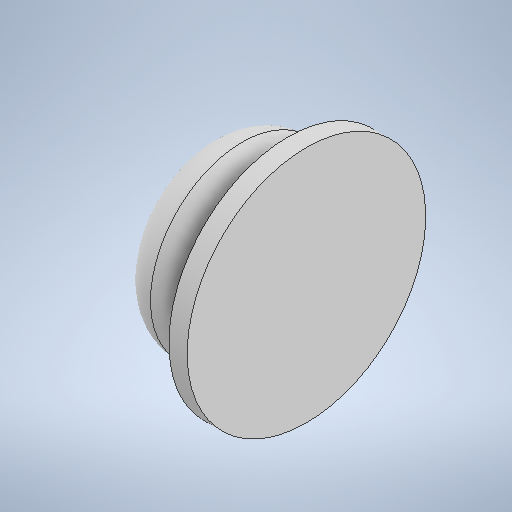
# Autodesk Inventor part: button
Saved by Autodesk Inventor 2025 (Build 290162000, 162)
## iProperties
Created: 2026-04-07
Part Number: button
Material: Generic
Document SubType Name: Modeling
Designer: Luca
Density: 1 g/cm^3
Appearance: Default
Author: Luca
Autodesk Inventor part; units mm, degrees
ref_plane "YZ Plane" through (0, 0, 0) normal (1, 0, 0) x (0, 1, 0)
ref_plane "XZ Plane" through (0, 0, 0) normal (0, 1, 0) x (-1, 0, 0)
ref_plane "XY Plane" through (0, 0, 0) normal (0, 0, 1) x (1, 0, 0)
derived "sk_reservoir.ipt"
sketch "button" plane through (-80, 0, 0) normal (1, 0, 0) x (0, 1, 0)
  line L0 (-57.9, 133.17) -> (-57.9, -125.8542)
  line L1 (-43.8, -4) -> (-49.9, -4)
  line L2 (-49.9, -4) -> (-49.9, 4)
  line L3 (-49.9, 4) -> (-43.8, 4)
  line L4 (-43.8, 4) -> (-43.8, -4)
  line L5 (-43.8, -1.25) -> (-49.9, -1.25)
  line L6 (-49.9, -1.25) -> (-49.9, 1.25)
  line L7 (-49.9, 1.25) -> (-43.8, 1.25)
  line L8 (-43.8, 1.25) -> (-43.8, -1.25)
  line L9 (-49.9, 0) -> (-0.1295, 0) construction
  line L10 (-132, 0) -> (302, 0) construction
  circle A0 centre (-46.85, 0) radius 6.5
  circle A1 centre (-46.85, 0) radius 6.25
  circle A2 centre (-46.85, 0) radius 5.25
  circle A3 centre (-46.85, 0) radius 5
  circle A4 centre (-46.85, 0) radius 8
  line L11 (-46.85, -8) -> (-57.9, -8)
  line L12 (-46.85, 8) -> (-57.9, 8)
  point P0 (0, 0)
  point P1 (-46.85, 4)
ref_plane "button_back" through (-77.5, 0, 0) normal (1, 0, 0) x (0, 1, 0)
ref_plane "hole" through (-80, 0, 0) normal (1, 0, 0) x (0, 1, 0)
extrude "Extrusion1" add sketch "button" along normal up to surface (1 mm away) from surface at 2.5 contours L1 A3 L4 | A3 L1 | L1 A3 L2 L5 L4 | L4 A3 | L1 L2 A3 | L5 L2 L7 L4 | A3 L2 | L7 L2 A3 L3 L4 | A3 L3 L4 | L2 L3 A3 | L3 A3 | A0 | A1 | A2
extrude "Extrusion2" add sketch "button" along normal up to surface (3.5 mm away) from surface at 0 contours A3 L1 | L1 A3 L2 L5 L4 | L4 A3 | L5 L2 L7 L4 | A3 L2 | L7 L2 A3 L3 L4 | L3 A3
extrude "Extrusion3" add sketch "button" against normal blind 2 contours A3 L1 | L1 A3 L2 L5 L4 | L4 A3 | L5 L2 L7 L4 | A3 L2 | L7 L2 A3 L3 L4 | L3 A3
fillet "Fillet1" radius 2 1 edges at (-82, -51.85, 0)
ref_plane "Work Plane20" through (-76.5, 0, 0) normal (1, 0, 0) x (0, 1, 0)
body "Solid1"
